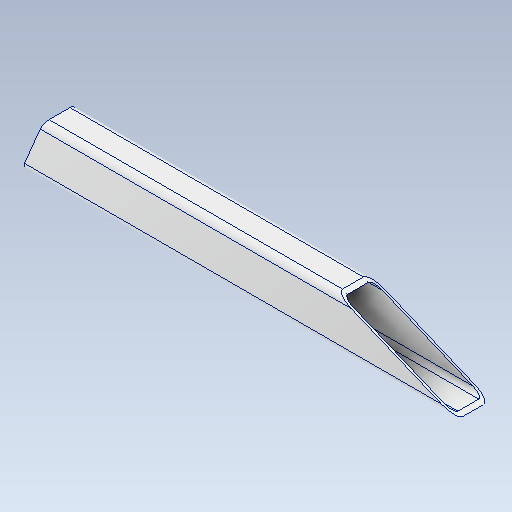
# Autodesk Inventor part: support 1
Saved by Autodesk Inventor 2021 (Build 250183000, 183)
## iProperties
Created: 2021-03-29
Part Number: support 1
Material: Aluminum 6061
Document SubType Name: Modeling
Designer: Work
Mass: 1079.47 g
Surface Area: 2545.07 cm^2
Volume: 399.804 cm^3
Density: 2.7 g/cm^3
Appearance: Aluminum - Flat
Author: Work
Autodesk Inventor part; units mm, degrees
ref_plane "YZ Plane" through (0, 0, 0) normal (1, 0, 0) x (0, 1, 0)
ref_plane "XZ Plane" through (0, 0, 0) normal (0, 1, 0) x (-1, 0, 0)
ref_plane "XY Plane" through (0, 0, 0) normal (0, 0, 1) x (1, 0, 0)
sketch "Sketch1" plane through (0, 0, 0) normal (1, 0, 0) x (0, 1, 0)
  line L0 (-28.575, 25.4) -> (28.575, 25.4)
  line L1 (38.1, 15.875) -> (38.1, -15.875)
  line L2 (28.575, -25.4) -> (-28.575, -25.4)
  line L3 (-38.1, -15.875) -> (-38.1, 15.875)
  line L4 (-38.1, 25.4) -> (38.1, -25.4) construction
  line L5 (38.1, 25.4) -> (-38.1, -25.4) construction
  arc A0 (38.1, 15.875) -> (28.575, 25.4) centre (28.575, 15.875) ccw
  arc A1 (-28.575, 25.4) -> (-38.1, 15.875) centre (-28.575, 15.875) ccw
  arc A2 (-38.1, -15.875) -> (-28.575, -25.4) centre (-28.575, -15.875) ccw
  arc A3 (28.575, -25.4) -> (38.1, -15.875) centre (28.575, -15.875) ccw
  line L6 (34.925, -15.875) -> (34.925, 15.875)
  arc A4 (34.925, 15.875) -> (28.575, 22.225) centre (28.575, 15.875) ccw
  line L7 (28.575, 22.225) -> (-28.575, 22.225)
  arc A5 (-28.575, 22.225) -> (-34.925, 15.875) centre (-28.575, 15.875) ccw
  line L8 (-34.925, 15.875) -> (-34.925, -15.875)
  arc A6 (-34.925, -15.875) -> (-28.575, -22.225) centre (-28.575, -15.875) ccw
  line L9 (-28.575, -22.225) -> (28.575, -22.225)
  arc A7 (28.575, -22.225) -> (34.925, -15.875) centre (28.575, -15.875) ccw
  point P0 (0, 0)
  dimension "d0" = 76.2
  dimension "d1" = 50.8
  dimension "d2" = 9.525
  dimension "d3" = 3.175
  constraints: 20 end point, 16 point on circle, 8 centre point, 8 point on line, 8 tangent, 4 parallel, 3 equal radius, 2 midpoint, 2 perpendicular, 1 horizontal, 7 other
  measures "d0" distance of L4.end L5.end
  measures "d1" distance of L5.start L4.end
  measures "d2" radius of A0
  measures "d3" distance between parallel lines of L1 L6
extrude "Extrusion1" add sketch "Sketch1" along normal blind 660.4
sketch "Sketch2" plane through (0, -28.575, 25.4) normal (0, 0, 1) x (1, 0, 0)
  line L0 (0, -9.525) -> (660.4, -9.525) projected
  line L1 (0, -9.525) -> (31.75, 66.675)
  line L2 (0, 66.675) -> (660.4, 66.675) projected
  line L3 (0, 57.15) -> (0, 0) projected
  line L4 (0, 57.15) -> (0, 66.675) projected
  line L5 (54.4286, 66.675) -> (0, 66.675)
  line L6 (0, 66.675) -> (0, -9.525)
  line L7 (660.4, -9.525) -> (477.52, 66.675)
  line L8 (477.52, 66.675) -> (660.4, 66.675)
  line L9 (660.4, 66.675) -> (660.4, -9.525)
  line L10 (0, 57.15) -> (660.4, 57.15) projected
  point P0 (0, 28.575)
  dimension "d6" = 22.62
  dimension "d7" = 22.62
  constraints: 12 end point, 3 perpendicular, 3 point on line, 1 horizontal
  measures "d6" angle of L3 L1
  measures "d7" angle of L0 L7
extrude "Extrusion2" cut sketch "Sketch2" against normal through all contours L6 L3 L10 L1 | L7 L10 L9 | L10 L4 L2 L1 | L7 L2 L9 L10
equation "\"d0\" = stockWidth"
equation "\"d1\" = stockHeight"
equation "\"d2\" = stockRad"
equation "\"d3\" = stockGuage"
equation "\"d4\" = sup1Len"
equation "\"d6\" = sup1Ang"
equation "\"d7\" = sup1Ang"
equation "\"height\" = 203.2"
equation "\"shaftDiam\" = 6.35"
equation "\"shaftSpace\" = 1.5875"
equation "\"stageSpace\" = 2.54"
equation "\"stageAngle\" = 15deg"
equation "\"stockHeight\" = 50.8"
equation "\"stockWidth\" = 76.2"
equation "\"stockRad\" = 9.525"
equation "\"stockGuage\" = 3.175"
equation "\"groundActu\" = 304.8"
equation "\"baseWidth\" = 1066.8"
equation "\"baseDepth\" = 254"
equation "\"capThickness\" = 3.175"
equation "\"sup1Len\" = 660.4"
equation "\"sup1Ang\" = 22.6199deg"
equation "\"supVertLen\" = 955.13561"
equation "\"sup2Ang\" = 8.959949deg"
equation "\"sup2Len\" = 2079.37366"
equation "\"supSideAng\" = 19.376933deg"
equation "\"supSideLen\" = 1531.12879"
equation "\"FlangeDiam\" = 12.7"
equation "\"bearingDiam\" = 9.5504"
equation "\"FlangeDepth\" = 1.5875"
equation "\"smallFilet\" = 0.39687"
equation "\"thickness\" = 12.7"
equation "\"ringDiam\" = 96.46608"
body "Solid1"
